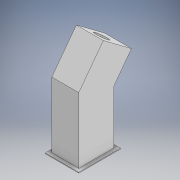
# Autodesk Inventor part: MountBase
Saved by Autodesk Inventor 2022 (Build 260153000, 153)
## iProperties
Created: 2021-04-30
Part Number: MountBase
Material: Generic
Document SubType Name: Modeling
Designer: Mick Veldhuis
Density: 1 g/cm^3
Appearance: Default
Author: Mick Veldhuis
Autodesk Inventor part; units mm, degrees
ref_plane "YZ Plane" through (0, 0, 0) normal (1, 0, 0) x (0, 1, 0)
ref_plane "XZ Plane" through (0, 0, 0) normal (0, 1, 0) x (-1, 0, 0)
sketch "Sketch1" plane through (0, 0, 0) normal (0, 1, 0) x (-1, 0, 0)
  line L0 (165, 215) -> (-165, 215)
  line L1 (-165, 215) -> (-165, -215)
  line L2 (-165, -215) -> (165, -215)
  line L3 (165, -215) -> (165, 215)
  line L4 (165, 215) -> (-165, -215) construction
  line L5 (-165, 215) -> (165, -215) construction
  point P0 (0, 0)
  dimension "d0" = 330
  dimension "d1" = 430
  constraints: 12 end point, 2 midpoint, 2 parallel, 1 horizontal, 1 perpendicular
  measures "d0" distance of L2.end L1.end
  measures "d1" distance of L1.end L0.end
extrude "Extrusion1" add sketch "Sketch1" along normal blind 816
move faces "Move1" translate (0, 400, 0) faces at (55, 816, 71.6667)
chamfer "Chamfer1" distance 300 angle 53.24 1 edges at (0, 1216, 215) measured on face at (55, 1216, 71.6667)
chamfer "Chamfer2" distance 130 angle 36.76 1 edges at (0, 1216, -215) measured on face at (55, 1216, -171.6667)
ref_plane "Work Plane1" through (165, 1216, -85) normal (0, 0.8011494, -0.5984644) x (1, 0, 0)
sketch "Sketch2" plane through (165, 1216, -85) normal (0, 0.8011494, -0.5984644) x (1, 0, 0)
  line L0 (-330, 0) -> (0, 0) projected
  line L1 (-330, 487.3879) -> (-330, 0) projected
  line L2 (0, 0) -> (-330, 0)
  line L3 (-330, 0) -> (-330, 430)
  line L4 (-330, 430) -> (0, 430)
  line L5 (0, 430) -> (0, 0)
  point P0 (-165, 659.6351)
  constraints: 8 end point, 2 parallel, 1 horizontal, 1 perpendicular, 1 point on line
extrude "Extrusion2" add sketch "Sketch2" against normal blind 358.4
sketch "Sketch3" plane through (-165, 1216, -85) normal (0, 0.8011494, -0.5984644) x (1, 0, 0)
  circle A0 centre (165, 180) radius 80
  point P0 (165, 659.6351)
  constraints: 1 centre point, 1 coincident
extrude "Extrusion3" cut sketch "Sketch3" against normal blind 400
sketch "Sketch4" plane through (0, 0, 0) normal (0, -1, 0) x (1, 0, 0)
  line L0 (165, 215) -> (-165, 215)
  line L1 (-165, 215) -> (-165, -215)
  line L2 (-165, -215) -> (165, -215)
  line L3 (165, -215) -> (165, 215)
  line L4 (165, 215) -> (-165, -215) construction
  line L5 (-165, 215) -> (165, -215) construction
  point P0 (0, 0)
  constraints: 12 end point, 2 midpoint, 2 parallel, 1 horizontal, 1 perpendicular
extrude "Extrusion4" cut sketch "Sketch4" against normal blind 10
sketch "Sketch5" plane through (0, 10, 0) normal (0, -1, 0) x (1, 0, 0)
  line L0 (205, 255) -> (-205, 255)
  line L1 (-205, 255) -> (-205, -255)
  line L2 (-205, -255) -> (205, -255)
  line L3 (205, -255) -> (205, 255)
  line L4 (205, 255) -> (-205, -255) construction
  line L5 (-205, 255) -> (205, -255) construction
  point P0 (0, 0)
  constraints: 12 end point, 2 midpoint, 2 parallel, 1 horizontal, 1 perpendicular
extrude "Extrusion5" add sketch "Sketch5" along normal blind 10
body "Solid1"
